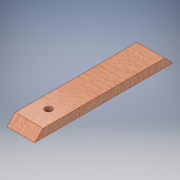
# Autodesk Inventor part: Front
Saved by Autodesk Inventor 2019.3 (Build 233278000, 278)
## iProperties
Created: 2019-01-12
Part Number: Front
Material: Holz (Eiche)
Document SubType Name: Modeling
Designer: Jonas
Density: 0.76 g/cm^3
Appearance: Weißeiche - natur - mittlerer Glanz
Author: Jonas
Autodesk Inventor part; units mm, degrees
ref_plane "YZ Plane" through (0, 0, 0) normal (1, 0, 0) x (0, 1, 0)
ref_plane "XZ Plane" through (0, 0, 0) normal (0, 1, 0) x (-1, 0, 0)
ref_plane "XY Plane" through (0, 0, 0) normal (0, 0, 1) x (1, 0, 0)
sketch "Skizze1" plane through (0, 0, 0) normal (0, 1, 0) x (-1, 0, 0)
  line L0 (35.9259, 133.0751) -> (-24.0741, 133.0751)
  line L1 (-24.0741, 133.0751) -> (-24.0741, -166.9249)
  line L2 (-24.0741, -166.9249) -> (35.9259, -166.9249)
  line L3 (35.9259, -166.9249) -> (35.9259, 133.0751)
  point P0 (0, 0)
  point P1 (5.9259, 83.0751)
  dimension "d0" = 60
  dimension "d1" = 300
  dimension "d24" = 30
  dimension "d25" = 50
  constraints: 8 end point, 2 parallel, 1 horizontal, 1 perpendicular
  measures "d0" distance of L0.start L0.end
  measures "d1" distance of L2.end L0.start
  measures "d24" distance from line of L1 point (5.926, 83.075)
  measures "d25" distance from line of L0 point (5.926, 83.075)
extrude "Extrusion1" add sketch "Skizze1" along normal blind 18
chamfer "Fase1" distance 18 angle 45 1 edges at (-5.9259, 18, 133.0751)
chamfer "Fase2" distance 18 angle 45 1 edges at (-5.9259, 18, -166.9249)
sketch "Skizze4" plane through (0, 0, 0) normal (0, -1, 0) x (1, 0, 0)
  line L0 (-35.9259, -166.9249) -> (-35.9259, 133.0751) projected
  line L1 (-35.9259, 133.0751) -> (24.0741, 133.0751) projected
  point P0 (0, 0)
  point P1 (-5.9259, 73.0751)
  dimension "d33" = 30
  dimension "d34" = 60
  measures "d33" distance from line of L0 point (-5.926, 73.075)
  measures "d34" distance from line of L1 point (-5.926, 73.075)
hole "Bohrung5" at (-5.9259, 0, 73.0751) direction (0, 1, 0) diameter 15 end through all
sketch "Skizze2" plane through (0, 18, 0) normal (0, 1, 0) x (1, 0, 0)
  point P0 (38.0741, -40.5751)
sketch "Skizze3" plane through (0, 18, 0) normal (0, 1, 0) x (1, 0, 0)
  point P0 (38.0741, 74.4249)
